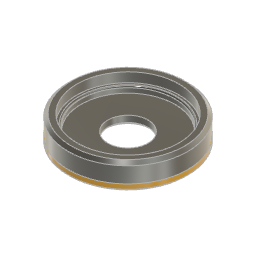
_32mm Magnet Base W_ Step and ring.4579ebb7-0c18-4f18-ad9a-c0d4c43d296b (Autodesk Fusion 360 design; units mm, degrees)
Autodesk Fusion 360 part; units mm, degrees
sketch "Sketch1" plane through (0, 0, 0) normal (0, 0, 1) x (1, 0, 0)
  circle A0 centre (0, 0) radius 16.25
  circle A1 centre (0, 0) radius 19
  circle A2 centre (0, 0) radius 6.4
  dimension "d1" = 32.5
  dimension "d2" = 38
  dimension "d3" = 12.8
  constraint coincident A0.centre A1.centre
  constraint concentric A0 A1
  constraint concentric A0 A2
  measures "d1" diameter of A0
  measures "d2" diameter of A1
  measures "d3" diameter of A2
extrude "Extrude1" add sketch "Sketch1" along normal blind 8 contours A1 makes body 1
extrude "Extrude2" add sketch "Sketch1" along normal blind 3 contours A0 bodies 1
chamfer "Chamfer1" distance 1 angle 45 1 edges at (-17.7142, -6.8707, 8) on bodies 1
chamfer "Chamfer2" distance 1 angle 45 1 edges at (-5.9669, 2.3143, 0) on bodies 1
sketch "Sketch2" plane through (0, 0, 3) normal (0, 0, 1) x (-1, 0, 0)
  circle A0 centre (0, 0) radius 6.4
  circle A1 centre (0, 0) radius 16.25
  circle A2 centre (0, 0) radius 15
  dimension "d10" = 30
  constraint coincident A0.centre A1.centre
  measures "d10" diameter of A2
extrude "Extrude3" add sketch "Sketch2" along normal blind 2 contours A1 bodies 1
fillet "Fillet1" radius 0.5 1 edges at (13.9849, -5.4242, 5) on bodies 1
chamfer "Chamfer3" distance 0.5 angle 45 1 edges at (-17.7142, -6.8707, 0) on bodies 1
extrude "Extrude4" cut sketch "Sketch1" along normal blind 2 contours A1 bodies 1
extrude "Extrude1'" add 1 faces at (17.9521, -1.7512, 2) along direction (0, 0, -1) blind 2 separate body on bodies 1 makes body 2 in component "Color Ring"
chamfer "Chamfer1'" distance 0.5 angle 45 1 edges at (-17.7142, 6.8707, 0) on bodies 2 in component "Color Ring"
component "Color Ring" placed x (1, 0, 0) y (0, 1, 0) z (0, 0, 1) at (0, 0, 0)
named bodies: "Single pole color Ring Base"
